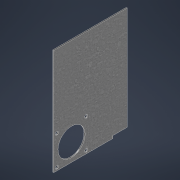
# Autodesk Inventor part: Soporte_Gearbox
Saved by Autodesk Inventor 2022 (Build 260153000, 153)
## iProperties
Part Number: Soporte_Gearbox
Material: Genérico
Document SubType Name: Modelado
Designer: seb_0
Appearance: Acero galvanizado
Author: seb_0
Autodesk Inventor part; units mm, degrees
ref_plane "Plano YZ" through (0, 0, 0) normal (1, 0, 0) x (0, 1, 0)
ref_plane "Plano XZ" through (0, 0, 0) normal (0, 1, 0) x (-1, 0, 0)
ref_plane "Plano XY" through (0, 0, 0) normal (0, 0, 1) x (1, 0, 0)
sketch "Boceto1" plane through (0, 0, 0) normal (1, 0, 0) x (0, 1, 0)
  circle A0 centre (0, 0) radius 37.5
  arc A1 (-49.5, -29.2575) -> (-49.5, 29.2575) centre (0, 0) ccw
  line L0 (0, 0) -> (-49.5, 0)
  circle A2 centre (40.6586, -40.6586) radius 4.5
  circle A3 centre (40.6586, 40.6586) radius 4.5
  circle A4 centre (-40.6586, 40.6586) radius 4.5
  circle A5 centre (-40.6586, -40.6586) radius 4.5
  line L1 (-40.6586, 40.6586) -> (0, 0)
  line L2 (0, 0) -> (40.6586, -40.6586)
  line L3 (-40.6586, -40.6586) -> (0, 0)
  line L4 (0, 0) -> (40.6586, 40.6586)
  line L5 (243, 49) -> (-82, 49)
  line L6 (-82, 49) -> (-82, -154)
  line L7 (-82, -154) -> (243, -154)
  line L8 (243, -154) -> (243, 49)
  circle A6 centre (230.5, 29) radius 4
  circle A7 centre (230.5, -29) radius 4
  circle A8 centre (-69.5, 29) radius 4
  circle A9 centre (-69.5, -29) radius 4
  line L9 (-82, -114) -> (-42, -114)
  line L10 (-42, -114) -> (-42, -154)
  dimension "d0" = 75
  dimension "d1" = 115
  dimension "d11" = 9
  dimension "d12" = 9
  dimension "d13" = 9
  dimension "d14" = 9
  dimension "d15" = 90
  dimension "d16" = 90
  dimension "d17" = 90
  dimension "d27" = 82
  dimension "d28" = 243
  dimension "d29" = 203
  dimension "d30" = 49
  dimension "d31" = 8
  dimension "d32" = 8
  dimension "d33" = 12.5
  dimension "d34" = 12.5
  dimension "d35" = 20
  dimension "d36" = 58
  dimension "d37" = 45
  dimension "d38" = 8
  dimension "d39" = 8
  dimension "d41" = 58
  dimension "d42" = 12.5
  dimension "d43" = 12.5
  dimension "d44" = 20
  dimension "d45" = 40
  dimension "d46" = 40
  constraints: 22 end point, 10 centre point, 6 point on circle, 3 horizontal, 2 coincident, 2 parallel, 2 perpendicular, 2 point on line
  measures "d0" diameter of A0
  measures "d1" diameter of A1
  measures "d11" diameter of A2
  measures "d12" diameter of A3
  measures "d13" diameter of A4
  measures "d14" diameter of A5
  measures "d15" angle of L2 L4
  measures "d16" angle of L3 L2
  measures "d17" angle of L1 L3
  measures "d27" distance from line of L6 point (0, 0)
  measures "d28" distance from line of L8 A0.centre
  measures "d29" distance between parallel lines of L7 L5
  measures "d30" distance from line of L5 point (0, 0)
  measures "d31" diameter of A6
  measures "d32" diameter of A7
  measures "d33" distance from line of L8 A6.centre
  measures "d34" distance from line of L8 A7.centre
  measures "d35" distance from line of L5 A6.centre
  measures "d36" distance of A7.centre A6.centre
  measures "d37" angle of L6 L4
  measures "d38" diameter of A8
  measures "d39" diameter of A9
  measures "d41" distance of A8.centre A9.centre
  measures "d42" distance from line of L6 A8.centre
  measures "d43" distance from line of L6 A9.centre
  measures "d44" distance from line of L5 A8.centre
  measures "d45" distance of L9.end L10.end
  measures "d46" distance of L9.start L9.end
extrude "Extrusión1" add sketch "Boceto1" along normal blind 2 contours A0 L4 A3 A1 A2 L2 | A0 L1 A4 A1 L5 A3 L4 | L2 A2 A1 A5 L3 A0 | A0 L3 A5 A1 A2 A3 L5 L8 L7 L10 L9 L6 A4 L1 | A6 | A7 | A8 | A9
sketch "Sketch2" plane through (2, 0, 0) normal (1, 0, 0) x (0, 0, -1)
  line L0 (-49, -82) -> (114, -82) projected
  line L1 (114, -82) -> (114, -42) projected
  line L2 (-49, -82) -> (114, -82)
  line L3 (114, -82) -> (114, -49)
  line L4 (114, -49) -> (-49, -49)
  line L5 (-49, -49) -> (-49, -82)
  line L6 (-64, -49) -> (46, -49) projected
  point P0 (0, 0)
  constraints: 8 end point, 2 parallel, 1 collinear, 1 horizontal, 1 perpendicular, 1 point on line
extrude "Extrusion2" cut sketch "Sketch2" against normal through all
